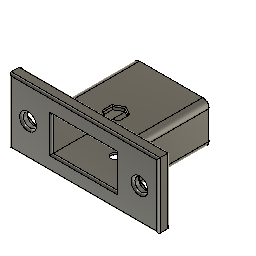
Powerpole Panel Mount (Autodesk Fusion 360 design; units mm, degrees)
Autodesk Fusion 360 part; units mm, degrees
sketch "Face" plane through (0, 0, 0) normal (0, 1, 0) x (1, 0, 0)
  line L0 (0, 0) -> (38.7, 0)
  line L1 (38.7, 0) -> (38.7, -17)
  line L2 (38.7, -17) -> (0, -17)
  line L3 (0, -17) -> (0, 0)
  line L4 (9.5, -13.85) -> (29.2, -13.85)
  line L5 (29.2, -13.85) -> (29.2, -3.15)
  line L6 (29.2, -3.15) -> (9.5, -3.15)
  line L7 (9.5, -3.15) -> (9.5, -13.85)
  line L8 (29.2, -3.15) -> (38.7, 0) construction
  line L9 (9.5, -13.85) -> (0, -17) construction
  line L10 (29.2, -13.85) -> (38.7, -17) construction
  line L11 (9.5, -3.15) -> (0, 0) construction
  line L12 (0, -17) -> (38.7, 0) construction
  line L13 (0, 0) -> (38.7, -17) construction
  circle A0 centre (4.85, -8.5) radius 1.7
  circle A1 centre (33.85, -8.5) radius 1.7
  line L14 (19.35, -8.5) -> (33.85, -8.5) construction
  line L15 (4.85, -8.5) -> (19.35, -8.5) construction
  line L16 (10.95, -12.9) -> (27.75, -12.9)
  line L17 (27.75, -12.9) -> (27.75, -4.1)
  line L18 (27.75, -4.1) -> (10.95, -4.1)
  line L19 (10.95, -4.1) -> (10.95, -12.9)
  line L20 (10.95, -4.1) -> (9.5, -3.15) construction
  line L21 (27.75, -4.1) -> (29.2, -3.15) construction
  line L22 (27.75, -12.9) -> (29.2, -13.85) construction
  line L23 (10.95, -12.9) -> (9.5, -13.85) construction
  point P0 (19.35, -8.5)
  dimension "d1" = 38.7
  dimension "d2" = 17
  dimension "d3" = 19.7
  dimension "d4" = 10.7
  dimension "d5" = 3.4
  dimension "d6" = 14.5
  dimension "d7" = 8.8
  dimension "d8" = 16.8
  constraint horizontal L0
  constraint vertical L1
  constraint horizontal L2
  constraint vertical L3
  constraint coincident L0.start L3.end
  constraint horizontal L4
  constraint vertical L5
  constraint horizontal L6
  constraint vertical L7
  constraint equal L10 L11
  constraint equal L8 L9
  constraint coincident L12 P0
  constraint coincident L13 P0
  constraint coincident P0 L14.start
  constraint coincident A1.centre L14.end
  constraint coincident A0.centre L15.start
  constraint horizontal L15
  constraint horizontal L14
  constraint equal A0 A1
  constraint equal L14 L15
  constraint horizontal L16
  constraint vertical L17
  constraint horizontal L18
  constraint vertical L19
  constraint equal L21 L23
  constraint equal L20 L22
  measures "d1" distance of L0.start L0.end
  measures "d2" distance of L0.start L2.end
  measures "d3" distance of L5.end L6.end
  measures "d4" distance of L4.start L6.end
  measures "d5" diameter of A0
  measures "d6" distance of A0.centre P0
  measures "d7" distance of L16.start L18.end
  measures "d8" distance of L17.end L18.end
extrude "Extrude1" add sketch "Face" against normal blind 3 contours L0 L1 L2 L3 | L4 L5 L6 L7
extrude "Extrude2" add sketch "Face" along normal blind 20 contours L4 L5 L6 L7
sketch "Connector Bolt Hole" plane through (0, 0, 13.85) normal (0, 0, 1) x (-1, 0, 0)
  line L0 (-9.5, 0) -> (-29.2, 0)
  line L1 (-29.2, 0) -> (-29.2, -20)
  line L2 (-29.2, -20) -> (-9.5, -20)
  line L3 (-9.5, -20) -> (-9.5, 0)
  circle A0 centre (-19.65, -5) radius 1.2
  line L4 (-19.65, 0) -> (-19.65, -5) construction
  line L5 (-29.2, -5) -> (-19.65, -5) construction
  line L6 (-19.65, -5) -> (-10.1, -5) construction
  line L7 (-10.1, -5) -> (-9.5, -5) construction
  point P0 (-19.65, -5)
  dimension "d13" = 2.4
  dimension "d15" = 5
  dimension "d68" = 0.6
  constraint coincident L0 L4.start
  constraint perpendicular L0 L4
  constraint coincident P0 A0.centre
  constraint coincident L1 L5.start
  constraint horizontal L5
  constraint perpendicular L4 L6
  constraint coincident L3 L7.end
  constraint perpendicular L3 L7
  constraint equal L5 L6
  measures "d13" diameter of A0
  measures "d15" distance of L4.start P0
  measures "d68" distance of L6.end L7.end
extrude "Extrude3" cut sketch "Connector Bolt Hole" against normal up to surface (10.7 mm away) contours A0
sketch "Panel Cut Corners" plane through (0, 20, 0) normal (0, 1, 0) x (-1, 0, 0)
  line L0 (-10.95, 12.9) -> (-10.95, 4.1)
  line L1 (-10.95, 4.1) -> (-27.75, 4.1)
  line L2 (-27.75, 4.1) -> (-27.75, 12.9)
  line L3 (-27.75, 12.9) -> (-10.95, 12.9)
  line L4 (-9.5, 3.15) -> (-9.5, 13.85)
  line L5 (-9.5, 13.85) -> (-29.2, 13.85)
  line L6 (-29.2, 13.85) -> (-29.2, 3.15)
  line L7 (-29.2, 3.15) -> (-9.5, 3.15)
  circle A0 centre (-27.55, 12.2) radius 1.65
  line L8 (-29.2, 13.85) -> (-19.65, 13.85)
  circle A1 centre (-11.15, 12.2) radius 1.65
  circle A2 centre (-11.15, 4.8) radius 1.65
  circle A3 centre (-27.55, 4.8) radius 1.65
  dimension "d70" = 3.3
  constraint tangent A0 L8
  constraint tangent L6 A0
  constraint equal A0 A1
  constraint equal A1 A2
  constraint equal A2 A3
  constraint tangent L8 A1
  constraint tangent L4 A1
  constraint tangent L4 A2
  constraint tangent L7 A2
  constraint tangent L7 A3
  constraint tangent L6 A3
  measures "d70" diameter of A0
extrude "Extrude13" cut sketch "Panel Cut Corners" against normal up to surface (20 mm away) contours L4 L5 A1 | L4 L7 A2 | L5 L6 A0 L8 | L6 L7 A3
fillet "Fillet4" radius 0.5 1 faces at (33.391, -3, 3.6349)
fillet "Fillet6" radius 0.5 1 edges at (20.7688, 5.4339, 3.15)
fillet "Fillet11" radius 0.5 4 edges at (19.35, 0, 0) (38.7, 0, 8.5) (19.35, 0, 17) (0, 0, 8.5)
fillet "Fillet12" radius 0.3 1 faces at (28.2333, 20, 7.2667)
sketch "Lower Grooves" plane through (0, 0, 12.9) normal (0, 0, -1) x (1, 0, 0)
  line L0 (27.75, 2.5) -> (10.95, 2.5)
  line L1 (10.95, 2.5) -> (10.95, -19.7)
  line L2 (27.75, -19.7) -> (27.75, 2.5)
  circle A0 centre (19.65, -5) radius 1.2
  line L3 (25.05, -20) -> (22.15, -20)
  line L4 (22.15, -20) -> (22.15, -6.5)
  line L5 (22.15, -6.5) -> (25.05, -6.5)
  line L6 (25.05, -6.5) -> (25.05, -20)
  line L7 (17.15, -20) -> (14.25, -20)
  line L8 (14.25, -20) -> (14.25, -6.5)
  line L9 (14.25, -6.5) -> (17.15, -6.5)
  line L10 (17.15, -6.5) -> (17.15, -20)
  line L11 (17.15, -6.5) -> (22.15, -6.5) construction
  line L12 (9.5, -20) -> (9.5, 0) construction
  line L13 (27.75, -19.7) -> (27.75, -20) construction
  line L14 (27.75, -20) -> (25.05, -20) construction
  line L15 (10.95, -19.7) -> (10.95, -20) construction
  line L16 (10.95, -20) -> (11.55, -20) construction
  line L17 (11.55, -20) -> (14.25, -20) construction
  line L18 (10.95, -19.7) -> (27.75, -19.7)
  dimension "d34" = 2.9
  dimension "d35" = 13.5
  dimension "d36" = 5
  dimension "d61" = 0.3
  dimension "d69" = 0.6
  constraint horizontal L3
  constraint vertical L4
  constraint horizontal L5
  constraint vertical L6
  constraint horizontal L7
  constraint vertical L8
  constraint horizontal L9
  constraint vertical L10
  constraint equal L5 L9
  constraint equal L4 L10
  constraint horizontal L11
  constraint coincident L2.start L13.start
  constraint perpendicular L13 L14
  constraint coincident L1.end L15.start
  constraint equal L13 L15
  constraint coincident L3.start L6.end
  constraint perpendicular L15 L16
  constraint perpendicular L8 L17
  constraint equal L14 L17
  constraint vertical L13
  measures "d34" distance of L4.end L5.end
  measures "d35" distance of L7.end L8.end
  measures "d36" distance of L4.end L9.end
  measures "d61" distance of L2.start L13.end
  measures "d69" distance of L15.end L16.end
extrude "Extrude5" add sketch "Lower Grooves" along normal blind 0.55 contours L4 L5 L6 L18 | L8 L9 L10 L18
sketch "Lower Groove Chamfer" plane through (25.05, 0, 0) normal (1, 0, 0) x (0, 1, 0)
  line L0 (19.7, 12.9) -> (6.5, 12.9)
  line L1 (6.5, 12.9) -> (6.5, 12.35)
  line L2 (6.5, 12.35) -> (19.7, 12.35)
  line L3 (7.05, 12.35) -> (6.5, 12.9)
  line L4 (7.05, 12.35) -> (6.5, 12.35)
  line L5 (6.5, 12.9) -> (6.5, 12.35)
  line L6 (19.7, 12.35) -> (19.7, 12.9)
  constraint coincident L2 L3.start
  constraint coincident L0.end L1.start
  constraint coincident L1.end L2.start
  constraint equal L4 L5
extrude "Extrude6" cut sketch "Lower Groove Chamfer" against normal up to surface (10.8 mm away) contours L1 L2 L3 L4 L5
fillet "Fillet7" radius 0.25 2 faces at (24.0833, 15.4833, 12.35) (16.1833, 11.2667, 12.35)
sketch "Side Groove" plane through (27.75, 0, 0) normal (-1, 0, 0) x (0, -1, 0)
  line L0 (2.5, 4.1) -> (2.5, 12.9)
  line L1 (2.5, 12.9) -> (-19.7, 12.9)
  line L2 (-19.7, 4.1) -> (2.5, 4.1)
  line L3 (-7.5, 7.05) -> (-20, 7.05)
  line L4 (-20, 7.05) -> (-20, 9.95)
  line L5 (-20, 9.95) -> (-7.5, 9.95)
  line L6 (-7.5, 9.95) -> (-7.5, 7.05)
  line L7 (-19.7, 4.1) -> (-20, 4.1) construction
  line L8 (-20, 4.1) -> (-20, 7.05) construction
  line L9 (-19.7, 12.9) -> (-20, 12.9) construction
  line L10 (-20, 12.9) -> (-20, 9.95) construction
  line L11 (-19.7, 12.9) -> (-19.7, 4.1)
  dimension "d52" = 12.5
  dimension "d53" = 2.9
  dimension "d60" = 0.3
  constraint horizontal L3
  constraint vertical L4
  constraint horizontal L5
  constraint vertical L6
  constraint coincident L2.start L7.start
  constraint perpendicular L2 L8
  constraint coincident L1.end L9.start
  constraint perpendicular L9 L10
  constraint equal L8 L10
  constraint equal L7 L9
  constraint coincident L3.end L4.start
  constraint coincident L4.end L5.start
  constraint horizontal L7
  measures "d52" distance of L4.end L5.end
  measures "d53" distance of L3.end L4.end
  measures "d60" distance of L1.end L9.end
extrude "Extrude14" add sketch "Side Groove" along normal blind 0.55 contours L3 L5 L6 L11
sketch "Side Groove Chamfer" plane through (0, 0, 7.05) normal (0, 0, -1) x (1, 0, 0)
  line L0 (27.75, -19.7) -> (27.75, -7.5)
  line L1 (27.75, -7.5) -> (27.2, -7.5)
  line L2 (27.2, -7.5) -> (27.2, -19.7)
  line L3 (27.2, -19.7) -> (27.75, -19.7)
  line L4 (27.75, -7.5) -> (27.2, -8.05)
  line L5 (27.2, -8.05) -> (27.2, -7.5)
  line L6 (27.2, -7.5) -> (27.75, -7.5)
  constraint coincident L0.end L1.start
  constraint coincident L2 L4.end
  constraint coincident L1.end L2.start
  constraint equal L5 L6
extrude "Extrude15" cut sketch "Side Groove Chamfer" against normal blind 2.9 contours L1 L2 L4 L5 L6
fillet "Fillet13" radius 0.25 1 faces at (27.2, 11.9333, 8.0167)
sketch "Panel Nut Recess" plane through (0, 0, 0) normal (0, 1, 0) x (-1, 0, 0)
  circle A0 centre (-4.85, 8.5) radius 1.7
  circle A1 centre (-33.85, 8.5) radius 1.7
  line L0 (-11.15, 3.15) -> (-27.55, 3.15)
  arc A2 (-29.2, 4.8) -> (-27.55, 3.15) centre (-27.55, 4.8) ccw
  line L1 (-29.2, 4.8) -> (-29.2, 12.2)
  arc A3 (-27.55, 13.85) -> (-29.2, 12.2) centre (-27.55, 12.2) ccw
  line L2 (-27.55, 13.85) -> (-11.15, 13.85)
  arc A4 (-9.5, 12.2) -> (-11.15, 13.85) centre (-11.15, 12.2) ccw
  line L3 (-9.5, 12.2) -> (-9.5, 4.8)
  arc A5 (-11.15, 3.15) -> (-9.5, 4.8) centre (-11.15, 4.8) ccw
  line L4 (-0.5, 16.5) -> (-38.2, 16.5)
  line L5 (-38.2, 16.5) -> (-38.2, 0.5)
  line L6 (-38.2, 0.5) -> (-0.5, 0.5)
  line L7 (-0.5, 0.5) -> (-0.5, 16.5)
  line L8 (-2.1, 6.9123) -> (-2.1, 10.0877)
  line L9 (-2.1, 10.0877) -> (-4.85, 11.6754)
  line L10 (-4.85, 11.6754) -> (-7.6, 10.0877)
  line L11 (-7.6, 10.0877) -> (-7.6, 6.9123)
  line L12 (-7.6, 6.9123) -> (-4.85, 5.3246)
  line L13 (-4.85, 5.3246) -> (-2.1, 6.9123)
  line L14 (-31.1, 6.9123) -> (-31.1, 10.0877)
  line L15 (-31.1, 10.0877) -> (-33.85, 11.6754)
  line L16 (-33.85, 11.6754) -> (-36.6, 10.0877)
  line L17 (-36.6, 10.0877) -> (-36.6, 6.9123)
  line L18 (-36.6, 6.9123) -> (-33.85, 5.3246)
  line L19 (-33.85, 5.3246) -> (-31.1, 6.9123)
  point P0 (-4.85, 8.5)
  point P1 (-33.85, 8.5)
  dimension "d83" = 2.75
  dimension "d84" = 2.75
  constraint coincident P0 A0.centre
  constraint coincident P1 A1.centre
  constraint parallel L5 L17
  constraint parallel L7 L11
  measures "d83" distance of P0 L13
  measures "d84" distance of P1 L19
sketch "Connector Nut Recess" plane through (0, 0, 13.85) normal (0, 0, 1) x (-1, 0, 0)
  line L0 (-17.6, -6.1836) -> (-17.6, -3.8164)
  line L1 (-17.6, -3.8164) -> (-19.65, -2.6329)
  line L2 (-19.65, -2.6329) -> (-21.7, -3.8164)
  line L3 (-21.7, -3.8164) -> (-21.7, -6.1836)
  line L4 (-21.7, -6.1836) -> (-19.65, -7.3671)
  line L5 (-19.65, -7.3671) -> (-17.6, -6.1836)
  line L6 (-27.55, 0) -> (-27.55, -19.7)
  point P0 (-19.65, -5)
  point P1 (-19.65, -5)
  dimension "d85" = 2.05
  constraint coincident P1 P0
  constraint parallel L3 L6
  measures "d85" distance of P1 L5
extrude "Extrude16" cut sketch "Panel Nut Recess" against normal blind 1.5 contours L8 L9 L10 L11 L12 L13 | L14 L15 L16 L17 L18 L19
extrude "Extrude17" cut sketch "Connector Nut Recess" against normal up to surface (0.95 mm away)
fillet "Fillet14" radius 0.25 12 edges at (35.225, 0, 6.1184) (32.475, 0, 6.1184) (31.1, 0, 8.5) (32.475, 0, 10.8816) (35.225, 0, 10.8816) (36.6, 0, 8.5) (6.225, 0, 6.1184) (3.475, 0, 6.1184) (2.1, 0, 8.5) (3.475, 0, 10.8816) (6.225, 0, 10.8816) (7.6, 0, 8.5)
fillet "Fillet16" radius 0.25 6 edges at (20.675, 3.2246, 13.85) (21.7, 5, 13.85) (20.675, 6.7754, 13.85) (18.625, 6.7754, 13.85) (17.6, 5, 13.85) (18.625, 3.2246, 13.85)
